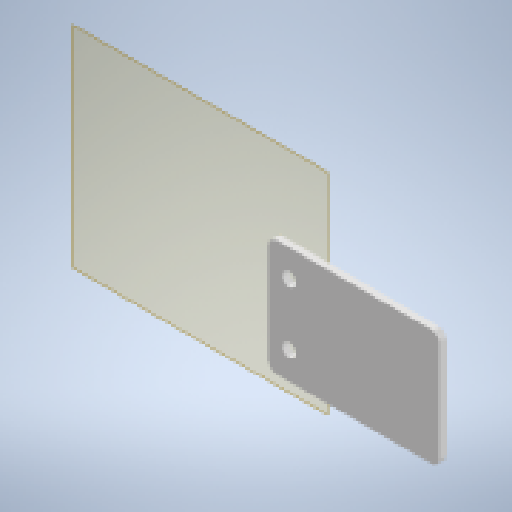
# Autodesk Inventor part: mocowanie silnika
Saved by Autodesk Inventor 2023 (Build 270158000, 158)
## iProperties
Created: 2023-04-14
Part Number: mocowanie silnika
Material: Ogólny
Document SubType Name: Modeling
Designer: krzys
Density: 1 g/cm^3
Appearance: Domyślna
Author: krzys
Autodesk Inventor part; units mm, degrees
ref_plane "YZ Plane" through (0, 0, 0) normal (1, 0, 0) x (0, 1, 0)
ref_plane "XZ Plane" through (0, 0, 0) normal (0, 1, 0) x (-1, 0, 0)
ref_plane "XY Plane" through (0, 0, 0) normal (0, 0, 1) x (1, 0, 0)
ref_plane "Płaszczyzna konstrukcyjna1" through (0, 0, 0) normal (0, 0, 1) x (1, 0, 0)
sketch "Szkic1" plane through (0, 0, 0) normal (0, 0, 1) x (1, 0, 0)
  circle A0 centre (85, 0) radius 5
  circle A1 centre (85, -45) radius 5
  line L0 (76, 20) -> (189, 20)
  line L1 (195, 14) -> (195, -59)
  line L2 (189, -65) -> (76, -65)
  line L3 (70, -59) -> (70, 14)
  arc A2 (70, -59) -> (76, -65) centre (76, -59) ccw
  arc A3 (76, 20) -> (70, 14) centre (76, 14) ccw
  arc A4 (189, -65) -> (195, -59) centre (189, -59) ccw
  arc A5 (195, 14) -> (189, 20) centre (189, 14) ccw
  point P0 (0, 0)
  point P1 (195, -65)
  point P2 (195, 20)
  point P3 (70, -65)
  dimension "d0" = 10
  dimension "d1" = 10
  dimension "d2" = 125
  dimension "d3" = 85
  dimension "d4" = 6
  constraints: 8 end point, 8 point on circle, 8 tangent, 6 centre point, 6 point on line, 3 equal radius, 2 parallel, 1 horizontal, 1 perpendicular
  measures "d0" diameter of A0
  measures "d1" diameter of A1
  measures "d2" distance of point (195, -65) point (70, -65)
  measures "d3" distance of point (195, 20) point (195, -65)
  measures "d4" radius of A2
extrude "Wyciągnięcie proste1" add sketch "Szkic1" along normal blind 5
